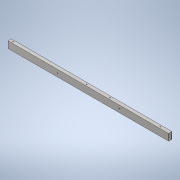
# Autodesk Inventor part: support-beam
Saved by Autodesk Inventor 2022 (Build 260153000, 153)
## iProperties
Created: 2021-12-06
Part Number: support-beam
Material: Generic
Document SubType Name: Modeling
Designer: Vedic
Density: 1 g/cm^3
Appearance: Default
Author: Vedic
Autodesk Inventor part; units mm, degrees
ref_plane "YZ Plane" through (0, 0, 0) normal (1, 0, 0) x (0, 1, 0)
ref_plane "XZ Plane" through (0, 0, 0) normal (0, 1, 0) x (-1, 0, 0)
ref_plane "XY Plane" through (0, 0, 0) normal (0, 0, 1) x (1, 0, 0)
sketch "Sketch1" plane through (0, 0, 0) normal (1, 0, 0) x (0, 1, 0)
  line L0 (-12.7, 12.7) -> (12.7, 12.7)
  line L1 (12.7, -12.7) -> (-12.7, -12.7)
  line L2 (12.7, 12.7) -> (25.4, 12.7)
  line L3 (25.4, 12.7) -> (25.4, -12.7)
  line L4 (25.4, -12.7) -> (12.7, -12.7)
  line L5 (-12.7, -12.7) -> (-25.4, -12.7)
  line L6 (-25.4, -12.7) -> (-25.4, 12.7)
  line L7 (-25.4, 12.7) -> (-12.7, 12.7)
  line L8 (22.86, -10.16) -> (22.86, 10.16)
  line L9 (22.86, 10.16) -> (12.7, 10.16)
  line L10 (12.7, 10.16) -> (-12.7, 10.16)
  line L11 (-12.7, 10.16) -> (-22.86, 10.16)
  line L12 (-22.86, 10.16) -> (-22.86, -10.16)
  line L13 (-22.86, -10.16) -> (-12.7, -10.16)
  line L14 (-12.7, -10.16) -> (12.7, -10.16)
  line L15 (12.7, -10.16) -> (22.86, -10.16)
  point P0 (0, 0)
  dimension "d1" = 25.4
  dimension "d14" = 25.4
  dimension "d15" = 50.8
  dimension "d16" = 12.7
  dimension "d17" = 2.54
  constraints: 32 end point, 8 perpendicular, 2 horizontal, 2 parallel, 2 point on line, 7 other
  measures "d1" distance between parallel lines of L0 L1
  measures "d14" distance from line of L3 point (0, 0)
  measures "d15" distance between parallel lines of L6 L3
  measures "d16" distance from line of L0 point (0, 0)
  measures "d17" distance between parallel lines of L3 L8
extrude "Extrusion1" add sketch "Sketch1" along normal blind 1219.2
sketch "Sketch3" plane through (0, -25.4, 12.7) normal (0, 0, 1) x (1, 0, 0)
  line L0 (0, 25.4) -> (1219.2, 25.4) construction
  line L1 (1219.2, 0) -> (1219.2, 50.8) construction
  line L2 (0, 50.8) -> (1219.2, 50.8) construction
  line L3 (609.6, 50.8) -> (609.6, 0) construction
  line L4 (0, 0) -> (1219.2, 0) construction
  circle A0 centre (843.28, 25.4) radius 3.175
  circle A1 centre (375.92, 25.4) radius 3.175
  dimension "d20" = 6.35
  dimension "d21" = 233.68
  dimension "d22" = 233.68
  constraints: 4 end point, 3 midpoint, 2 centre point, 2 point on line, 1 equal radius
  measures "d20" diameter of A1
  measures "d21" distance from line of L3 A1.centre
  measures "d22" distance from line of L3 A0.centre
extrude "Extrusion3" cut sketch "Sketch3" against normal through all
sketch "Sketch4" plane through (0, 25.4, 12.7) normal (0, 1, 0) x (1, 0, 0)
  line L0 (1219.2, 0) -> (1219.2, 25.4) projected
  line L1 (1219.2, 12.7) -> (0, 12.7) construction
  circle A0 centre (25.4, 12.7) radius 3.175
  circle A1 centre (1143, 12.7) radius 3.175
  line L2 (0, 25.4) -> (1219.2, 25.4) construction
  line L3 (609.6, 25.4) -> (609.6, 0) construction
  line L4 (0, 0) -> (1219.2, 0) construction
  line L5 (0, 25.4) -> (0, 0) projected
  circle A2 centre (762, 12.7) radius 3.175
  circle A3 centre (584.2, 12.7) radius 3.175
  dimension "d25" = 6.35
  dimension "d32" = 25.4
  dimension "d33" = 76.2
  dimension "d34" = 152.4
  dimension "d35" = 381
  dimension "d36" = 635
  constraints: 4 centre point, 4 end point, 4 point on line, 3 equal radius, 3 midpoint, 1 horizontal
  measures "d25" diameter of A0
  measures "d32" distance from line of L5 A0.centre
  measures "d33" distance from line of A1.centre L0
  measures "d34" distance from line of L3 A2.centre
  measures "d35" distance of A1.centre A2.centre
  measures "d36" distance of L1.start A3.centre
extrude "Extrusion4" cut sketch "Sketch4" against normal through all
equation "\"d14\" = 0.5 * d15"
equation "\"d16\" = 0.5 * d1"
equation "\"d22\" = d21"
body "Solid1"
